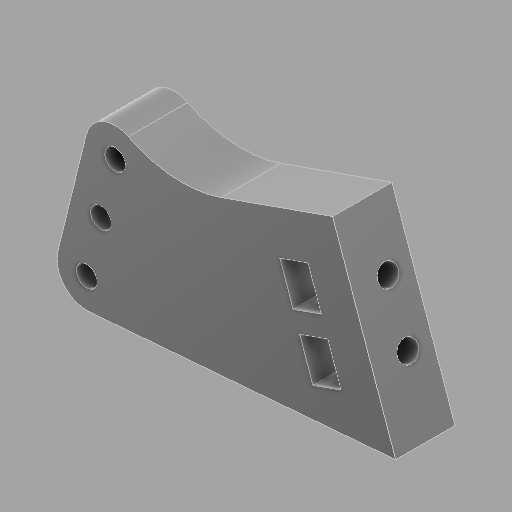
# Autodesk Inventor part: AngleSupport
Saved by Autodesk Inventor 2026.1 (Build 301233000, 233)
## iProperties
Created: 2025-09-14
Part Number: AngleSupport
Material: Plastic, Opaque Black
Document SubType Name: Modeling
Designer: Teddy
Density: 0.952 g/cm^3
Appearance: Smooth - Black
Author: Teddy
Autodesk Inventor part; units mm, degrees
ref_plane "YZ Plane" through (0, 0, 0) normal (1, 0, 0) x (0, 1, 0)
ref_plane "XZ Plane" through (0, 0, 0) normal (0, 1, 0) x (-1, 0, 0)
ref_plane "XY Plane" through (0, 0, 0) normal (0, 0, 1) x (1, 0, 0)
ref_plane "Work Plane1" through (-2.4446, 6.0882, -1.5875) normal (0, 0, -1) x (-0.2390086, -0.9710174, 0)
sketch "Sketch1" plane through (-2.4446, 6.0882, -1.5875) normal (0, 0, -1) x (-0.2390086, -0.9710174, 0)
  circle A0 centre (85.725, 10.3187) radius 2.1844
  circle A1 centre (98.425, 10.3187) radius 2.1844
  circle A2 centre (73.025, 10.3187) radius 2.1844
  line L0 (73.025, 10.3187) -> (98.425, 10.3187) construction
  line L1 (73.025, 3.9687) -> (98.425, 3.9687) construction
  line L2 (98.425, 16.6687) -> (73.025, 16.6687)
  arc A3 (73.025, 16.6687) -> (66.8404, 8.879) centre (73.025, 10.3187) ccw
  arc A4 (98.425, 3.9687) -> (104.4463, 8.3022) centre (98.425, 10.3187) ccw construction
  line L3 (73.025, 3.9687) -> (63.3473, -10.8009) construction
  arc A5 (63.3473, -10.8009) -> (66.8404, 8.879) centre (42.1019, 3.1199) ccw
  line L4 (58.7003, -37.8788) -> (62.3545, -40.2732)
  line L5 (69.323, -44.8393) -> (72.9773, -47.2337)
  line L6 (63.3473, -10.8009) -> (49.5384, -31.8756)
  arc A6 (66.8404, 8.879) -> (73.025, 3.9687) centre (73.025, 10.3187) ccw construction
  arc A7 (104.4463, 8.3022) -> (98.425, 16.6687) centre (98.425, 10.3187) ccw
  line L7 (69.2168, -44.7697) -> (68.3468, -46.0975)
  line L8 (73.0835, -47.3033) -> (72.2134, -48.6311)
  line L9 (68.7818, -45.4336) -> (72.6485, -47.9672) construction
  line L10 (70.7151, -46.7004) -> (77.6756, -36.0777) construction
  line L11 (60.5274, -39.076) -> (67.0528, -29.1172) construction
  line L12 (65.2343, -24.1298) -> (61.7541, -29.4412)
  line L13 (61.7541, -29.4412) -> (68.8713, -34.1047)
  line L14 (68.8713, -34.1047) -> (72.3515, -28.7933)
  line L15 (72.3515, -28.7933) -> (65.2343, -24.1298)
  line L16 (65.2343, -24.1298) -> (68.8713, -34.1047) construction
  line L17 (61.7541, -29.4412) -> (72.3515, -28.7933) construction
  line L18 (75.857, -31.0902) -> (72.3768, -36.4016)
  line L19 (72.3768, -36.4016) -> (79.4941, -41.0651)
  line L20 (79.4941, -41.0651) -> (82.9743, -35.7537)
  line L21 (82.9743, -35.7537) -> (75.857, -31.0902)
  line L22 (75.857, -31.0902) -> (79.4941, -41.0651) construction
  line L23 (72.3768, -36.4016) -> (82.9743, -35.7537) construction
  line L24 (181.7138, -118.4821) -> (130.5502, -84.9577) construction
  line L25 (49.5384, -31.8756) -> (83.5311, -54.149)
  line L26 (83.5311, -54.149) -> (104.4463, 8.3022)
  point P0 (85.725, 10.3187)
  point P1 (58.7003, -37.8788)
  point P2 (62.3545, -40.2732)
  point P3 (72.9773, -47.2337)
  dimension "d5" = 12.7
  dimension "d6" = 25.4
  dimension "d9" = 12.7
  dimension "d11" = 12.7
  dimension "d12" = 8.509
  dimension "d13" = 8.509
  dimension "d14" = 6.35
  dimension "d15" = 6.35
  dimension "d16" = 40.64
  constraints: 56 end point, 12 tangent, 10 point on circle, 9 midpoint, 8 centre point, 6 parallel, 6 perpendicular, 2 collinear, 1 horizontal, 1 point on line, 21 other
  measures "d5" diameter of A4
  measures "d6" radius of A5
  measures "d9" distance of L10.start L10.end
  measures "d11" distance between parallel lines of L10 L11
  measures "d12" distance of L13.end L12.end
  measures "d13" distance of L19.end L18.end
  measures "d14" distance of L18.start L18.end
  measures "d15" distance of L13.end L14.end
  measures "d16" distance of L6.end L25.end
ref_plane "Work Plane3" through (-129.6539, 63.7298, -14.2875) normal (0, 0, -1) x (-0.5480654, 0.8364355, 0)
extrude "Extrusion1" add sketch "Sketch1" along normal up to surface (12.7 mm away)
sketch "Sketch2" plane through (16.667, -49.633, -14.2875) normal (0.9431858, 0.3322658, 0) x (0, 0, 1)
  circle A0 centre (5.1816, 25.8379) radius 2.1844 projected
  circle A1 centre (5.1816, 13.1379) radius 2.1844 projected
  point P0 (14.2875, -52.351)
extrude "Extrusion2" cut sketch "Sketch2" against normal blind 12.7
body "Solid1"
